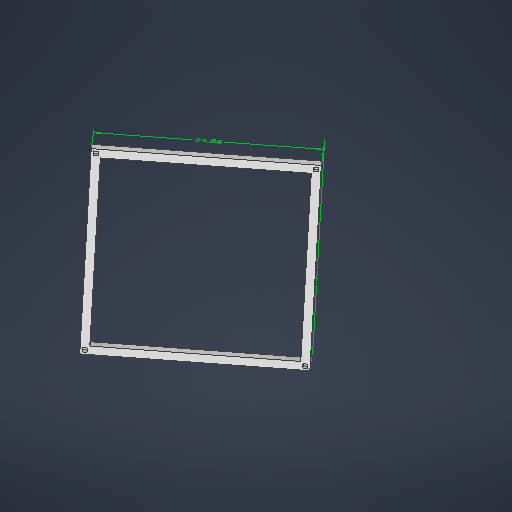
# Autodesk Inventor part: Pieza idividula 2
Saved by Autodesk Inventor 2027 (Build 310192000, 192)
## iProperties
Created: 2026-04-14
Part Number: Pieza idividula 2
Material: Genérico
Document SubType Name: Modeling
Designer: leand
Density: 1 g/cm^3
Appearance: Valor por defecto
Author: leand
Autodesk Inventor part; units mm, degrees
ref_plane "YZ Plane" through (0, 0, 0) normal (1, 0, 0) x (0, 1, 0)
ref_plane "XZ Plane" through (0, 0, 0) normal (0, 1, 0) x (-1, 0, 0)
ref_plane "XY Plane" through (0, 0, 0) normal (0, 0, 1) x (1, 0, 0)
sketch "Boceto1" plane through (0, 0, 0) normal (0, 1, 0) x (-1, 0, 0)
  line L0 (2.2316, -6.4309) -> (2.2316, -30.4309)
  line L1 (2.2316, -30.4309) -> (26.2316, -30.4309)
  line L2 (26.2316, -30.4309) -> (26.2316, -6.4309)
  line L3 (26.2316, -6.4309) -> (2.2316, -6.4309)
  line L4 (25.2316, -29.4309) -> (3.2316, -29.4309)
  line L5 (3.2316, -7.4309) -> (3.2316, -29.4309)
  line L6 (3.2316, -7.4309) -> (25.2316, -7.4309)
  line L7 (25.2316, -29.4309) -> (25.2316, -7.4309)
  point P0 (0, 0)
  dimension "d0" = 24
  dimension "d1" = 24
  constraints: 16 end point, 3 perpendicular, 1 vertical
  measures "d0" distance of L0.start L0.end
  measures "d1" distance of L0.end L1.end
extrude "Extrusión1" add sketch "Boceto1" along normal mid plane 1
sketch "Boceto2" plane through (0, 0.5, 0) normal (0, 1, 0) x (1, 0, 0)
  line L0 (-26.2316, 6.4309) -> (-2.2316, 6.4309) projected
  line L1 (-3.2316, 7.4309) -> (-25.2316, 7.4309) projected
  line L2 (-2.4816, 7.1809) -> (-2.4816, 6.6809)
  line L3 (-2.4816, 6.6809) -> (-2.9816, 6.6809)
  line L4 (-2.9816, 6.6809) -> (-2.9816, 7.1809)
  line L5 (-2.9816, 7.1809) -> (-2.4816, 7.1809)
  line L6 (-25.2316, 29.4309) -> (-3.2316, 29.4309) projected
  line L7 (-2.9816, 29.6809) -> (-2.4816, 29.6809)
  line L8 (-2.4816, 29.6809) -> (-2.4816, 30.1809)
  line L9 (-2.4816, 30.1809) -> (-2.9816, 30.1809)
  line L10 (-2.9816, 30.1809) -> (-2.9816, 29.6809)
  line L11 (-2.2316, 30.4309) -> (-26.2316, 30.4309) projected
  line L12 (-25.9816, 30.1809) -> (-25.9816, 29.6809)
  line L13 (-25.9816, 29.6809) -> (-25.4816, 29.6809)
  line L14 (-25.4816, 29.6809) -> (-25.4816, 30.1809)
  line L15 (-25.4816, 30.1809) -> (-25.9816, 30.1809)
  line L16 (-26.2316, 30.4309) -> (-26.2316, 6.4309) projected
  line L17 (-25.9816, 7.1809) -> (-25.9816, 6.6809)
  line L18 (-25.9816, 6.6809) -> (-25.4816, 6.6809)
  line L19 (-25.4816, 6.6809) -> (-25.4816, 7.1809)
  line L20 (-25.4816, 7.1809) -> (-25.9816, 7.1809)
  point P0 (0, 0)
  constraints: 32 end point, 6 perpendicular, 3 horizontal
extrude "Extrusión2" cut sketch "Boceto2" against normal blind 0.5
